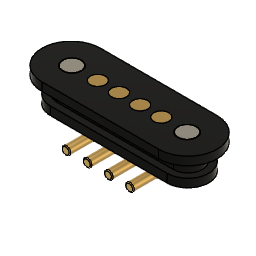
5358 Mag Connector (4-pin, Right Angle, Pads) (Autodesk Fusion 360 design; units mm, degrees)
Autodesk Fusion 360 part; units mm, degrees
sketch "Profile" plane through (0, 0, 0) normal (0, 0, 1) x (1, 0, 0)
  line L0 (0, 3.5) -> (0, -3.5) construction
  circle A0 centre (-6.91, 0) radius 1.125
  circle A1 centre (-3.81, 0) radius 0.45
  circle A2 centre (-1.27, 0) radius 0.45
  circle A3 centre (1.27, 0) radius 0.45
  circle A4 centre (6.91, 0) radius 1.125
  circle A5 centre (-3.81, 0) radius 0.5
  circle A6 centre (-3.81, 0) radius 0.9
  circle A7 centre (-1.27, 0) radius 0.5
  circle A8 centre (-1.27, 0) radius 0.9
  circle A9 centre (1.27, 0) radius 0.5
  circle A10 centre (1.27, 0) radius 0.9
  circle A11 centre (-3.81, 0) radius 0.575
  circle A12 centre (-1.27, 0) radius 0.575
  circle A13 centre (1.27, 0) radius 0.575
  circle A14 centre (3.81, 0) radius 0.45
  circle A15 centre (3.81, 0) radius 0.5
  circle A16 centre (3.81, 0) radius 0.9
  circle A17 centre (3.81, 0) radius 0.575
  line L1 (-10.5, 0) -> (10.5, 0) construction
  line L2 (-7, 1.725) -> (-7, -1.725) construction
  line L3 (-7, 2.5) -> (-7, -2.5) construction
  line L4 (0, 3.5) -> (-7, 3.5)
  line L5 (0, -3.5) -> (-7, -3.5)
  line L6 (-7, 3.5) -> (-7, -3.5) construction
  arc A18 (-7, 3.5) -> (-7, -3.5) centre (-7, 0) ccw
  arc A19 (-7, 2.5) -> (-7, -2.5) centre (-7, 0) ccw
  arc A20 (-7, 1.725) -> (-7, -1.725) centre (-7, 0) ccw
  line L7 (-7, 2.5) -> (0, 2.5)
  line L8 (-7, 1.725) -> (0, 1.725)
  line L9 (-7, -1.725) -> (0, -1.725)
  line L10 (-7, -2.5) -> (0, -2.5)
  line L11 (0, 3.5) -> (7, 3.5)
  arc A21 (7, -3.5) -> (7, 3.5) centre (7, 0) ccw
  line L12 (0, -3.5) -> (7, -3.5)
  line L13 (7, -2.5) -> (0, -2.5)
  arc A22 (7, -2.5) -> (7, 2.5) centre (7, 0) ccw
  line L14 (7, -1.725) -> (0, -1.725)
  arc A23 (7, -1.725) -> (7, 1.725) centre (7, 0) ccw
  line L15 (7, 1.725) -> (0, 1.725)
  line L16 (7, 2.5) -> (0, 2.5)
  line L17 (-1.25, 1.9) -> (1.25, 1.9)
  line L18 (-1.25, 1.9) -> (-1.25, 2.5)
  line L19 (1.25, 1.9) -> (1.25, 2.5)
  line L20 (-1, 3.375) -> (1, 3.375)
  line L21 (-1.875, 2.5) -> (-1, 3.375)
  line L22 (1, 3.375) -> (1.875, 2.5)
  dimension "d1" = 2.25
  dimension "d10" = 0.9
  dimension "d11" = 3.1
  dimension "d16" = 2.54
  dimension "d17" = 0
  dimension "d19" = 1
  dimension "d20" = 1.8
  dimension "d45" = 1.15
  dimension "d104" = 13.82
  dimension "d105" = 7
  dimension "d106" = 21
  dimension "d107" = 3.45
  dimension "d108" = 5
  dimension "d119" = 2.5
  dimension "d120" = 0.6
  dimension "d121" = 2
  dimension "d122" = 3.75
  dimension "d132" = 45
  constraint vertical L0
  constraint symmetric L0 A0 A4
  constraint concentric A1 A5
  constraint concentric A1 A6
  constraint midpoint origin L0
  constraint concentric A6 A11
  constraint horizontal L1
  constraint midpoint origin L1
  constraint perpendicular L1 L2
  constraint symmetric L1 L2.start L2.end
  constraint vertical L3
  constraint symmetric L1 L3.start L3.end
  constraint vertical L6
  constraint horizontal L4
  constraint horizontal L5
  constraint midpoint L6 A18.centre
  constraint coincident L1.start A18
  constraint midpoint L3 A18.centre
  constraint midpoint L2 A18.centre
  constraint collinear L3 L6
  constraint collinear L2 L6
  constraint coincident L0 L7.end
  constraint tangent A19 L7
  constraint coincident L0 L8.end
  constraint tangent A20 L8
  constraint coincident L0 L9.end
  constraint tangent A20 L9
  constraint coincident L0 L10.end
  constraint tangent A19 L10
  constraint symmetric L4.start L0 L11.start
  constraint symmetric L5.start L0 L12.start
  constraint symmetric L0 L2.start A23.end
  constraint symmetric L0 L2.end L14.start
  constraint symmetric L0 L3.start A22.end
  constraint symmetric L0 L3.end L13.start
  constraint symmetric L0 L4.end L11.end
  constraint symmetric L0 L5.end A21.start
  constraint symmetric L0 A18 A21
  constraint symmetric L0 A19 A22
  constraint symmetric L0 A20 A23
  constraint symmetric L0 L7.end L16.end
  constraint symmetric L0 L8.end L15.end
  constraint symmetric L0 L9.end L14.end
  constraint symmetric L0 L10.end L13.end
  constraint coincident A0.centre L1
  constraint coincident A1.centre L1
  constraint horizontal L17
  constraint symmetric L0 L17.start L17.end
  constraint coincident L7 L18.end
  constraint perpendicular L7 L18
  constraint coincident L16 L19.end
  constraint perpendicular L16 L19
  constraint horizontal L20
  constraint symmetric L0 L20.start L20.end
  constraint coincident L7 L21.start
  constraint coincident L16 L22.end
  constraint symmetric L0 L21.start L22.end
  measures "d1" diameter of A0
  measures "d10" diameter of A1
  measures "d11" distance of A0.centre A1.centre
  measures "d19" diameter of A5
  measures "d20" diameter of A6
  measures "d45" diameter of A11
  measures "d104" distance of A0.centre A4.centre
  measures "d105" distance of L0.start L0.end
  measures "d106" distance of L1.start L1.end
  measures "d107" distance of L2.start L2.end
  measures "d108" distance of L3.start L3.end
  measures "d119" distance of L17.start L17.end
  measures "d120" distance of L17.end L19.end
  measures "d121" distance of L20.start L20.end
  measures "d122" distance of L21.start L22.end
  measures "d132" angle of L20 L21
extrude "Extrude - Housing" add sketch "Profile" along normal blind 4 contours A20 L8 L9 L14 A23 L15 makes body 1
extrude "Extrude - Housing Flange" add sketch "Profile" against normal blind 1 from surface at 4 contours L4 L5 A18 L11 A21 L12 | A19 L7 L10 L13 A22 L16 L17 L18 L19 | L7 L16 L20 L21 L22 | L7 L16 L17 L18 L19 bodies 1
extrude "Extrude - Housing Flange Base" add sketch "Profile" against normal blind 0.65 from surface at 3 contours A19 L7 L10 L13 A22 L16 L17 L18 L19 | L7 L16 L17 L18 L19 bodies 1
extrude "Extrude - Housing Bottom Flange" add sketch "Profile" along normal blind 1 contours A19 L7 L10 L13 A22 L16 L17 L18 L19 | L7 L16 L17 L18 L19 bodies 1
extrude "Extrude - Housing Pin Clearance" add sketch "Profile" along normal up to surface (3.8 mm away) from surface at 0.2 contours A6 | A8 | A10 | A16 bodies 1
copy_body "Body->Comp1" bodies 1 removing the originals makes body 2 in component "Housing"
extrude "Extrude - Magnets" add sketch "Profile" along normal blind 4 separate body contours A0 | A4 makes body 3 at (-5.7906, -0.112, 1.3333) makes body 4 at (8.0336, -0.0561, 2.6667)
copy_body "Body->Comp2" bodies 3 removing the originals makes body 5 in component "Magnet"
fillet "Fillet - Magnets" radius 0.05 1 edges at (5.8611, -0.4068, 4) on bodies 4
fillet "Fillet1" radius 0.05 1 edges at (-7.9589, -0.4068, 4) on bodies 5 in component "Magnet"
fillet "Fillet1'" [no effect] in component "Housing"
fillet "Fillet3" radius 0.2 1 edges at (5.8611, -0.4068, 0) on bodies 4
fillet "Fillet2" radius 0.2 1 edges at (-7.9589, -0.4068, 0) on bodies 5 in component "Magnet"
copy_body "CutPasteBodies1" bodies 4 removing the originals makes body 6 in component "Magnet"
extrude "Extrude - Pin Bottom" add sketch "Profile" against normal blind 0.1 separate body contours A1 | A5 makes body 7 in component "Pins"
extrude "Extrude - Pin Base" add sketch "Profile" along normal blind 0.2 contours A1 | A5 | A6 | A11 bodies 7 in component "Pins"
extrude "Extrude - Pin Body" add sketch "Profile" along normal blind 3.6 contours A5 | A11 bodies 7 in component "Pins"
ref_plane "WorkPlane1" through (-1.27, 0, 0) normal (1, 0, 0) x (0, 1, 0)
sketch "Pin Right Angle Profile" plane through (-1.27, 0, 0) normal (1, 0, 0) x (0, 1, 0)
  line L0 (0, 0) -> (0, -0.65)
  line L1 (0, -0.65) -> (-0.75, -0.65) construction
  line L2 (-0.75, -0.65) -> (-0.75, -1.4) construction
  line L3 (-0.75, -1.4) -> (-3.85, -1.4)
  arc A0 (-0.75, -1.4) -> (0, -0.65) centre (-0.75, -0.65) ccw
  dimension "d94" = 0.75
  dimension "d109" = 3.85
  dimension "d110" = 0.65
  constraint vertical L0
  constraint perpendicular L0 L1
  constraint perpendicular L1 L2
  constraint perpendicular L2 L3
  constraint coincident L0.start origin
  constraint coincident L1.end L2.start
  constraint coincident L2.end L3.start
  measures "d94" distance of L0.end L1.end
  measures "d109" distance of L0 L3.end
  measures "d110" distance of L0.start L1
sweep "Sweep - Pin Right Angle" add 1 faces at (-3.9139, -0.1303, -0.1) path "Pin Right Angle Profile" along L0 A0 L3 on bodies 7 bodies 7 in component "Pins"
fillet "Fillet - Pin" radius 0.1 1 edges at (-4.2762, -3.85, -1.5808) on bodies 7 in component "Pins"
extrude "Extrude - Pad Clearance" cut sketch "Profile" against normal up to surface (0.4 mm away) from surface at 4 contours A6 bodies 2 in component "Housing"
pattern_linear "R-Pattern - Pad Clearance" count 4 spacing 2.54 along (1, 0, 0) of "Extrude - Pad Clearance" in component "Housing"
extrude "Extrude - Pad" add sketch "Profile" along normal up to surface (0.4 mm away) from surface at 3.6 contours A1 | A5 | A6 | A11 bodies 7 in component "Pins"
pattern_linear "R-Pattern - Pads" count 4 spacing 2.54 along (1, 0, 0) of bodies 7 makes body 8 at (-0.6979, 0.0573, 1.3333) makes body 9 at (1.8421, 0.0573, 1.3333) makes body 10 at (4.3821, 0.0573, 1.3333) in component "Pins"
extrude "Extrude2" add sketch "Profile" against normal blind 0.5 from surface at 3 contours L7 L16 L20 L21 L22 bodies 2 in component "Housing"
extrude "Extrude3" add sketch "Profile" against normal blind 0.5 contours L7 L16 L17 L18 L19 bodies 2 in component "Housing"
chamfer "Chamfer1" distance 0.3 distance2 0.5 1 edges at (0, 1.9, -0.5) measured on face at (-0.4167, 2.3, -0.5) on bodies 2 in component "Housing"
chamfer "Chamfer2" distance 0.2 distance2 0.5 2 edges at (-1.25, 2.35, -0.5) (1.25, 2.35, -0.5) measured on face at (-0.4167, 2.4, -0.5) measured on face at (-0.4167, 2.4, -0.5) on bodies 2 in component "Housing"
component "Housing" placed x (1, 0, 0) y (0, 1, 0) z (0, 0, 1) at (0, 0, 0)
component "Magnet" placed x (1, 0, 0) y (0, 1, 0) z (0, 0, 1) at (0, 0, 0)
component "Pins" placed x (1, 0, 0) y (0, 1, 0) z (0, 0, 1) at (0, 0, 0)
equation "d14 = 4"
equation "d89 = -( ( 2.54 * 0.5 ) * 1 mm )"
equation "d104 = ( d11 * 2 ) + ( d16 * ( d14 - 1 ) )"
named bodies: "Housing", "Magnet", "Magnet (1)", "Magnet (2)", "Pin (1)", "Pin (2)", "Pin (3)", "Pin (1) (1)"
